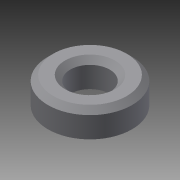
# Autodesk Inventor part: SpoolHandle-stop1
Saved by Autodesk Inventor 2014 (Build 180170000, 170)
## iProperties
Created: 2014-04-05
Part Number: SpoolHandle-stop1
Material: Generic
Document SubType Name: Modeling
Designer: Krzysiek
Density: 1 g/cm^3
Appearance: Default
Author: Krzysiek
Autodesk Inventor part; units mm, degrees
ref_plane "YZ Plane" through (0, 0, 0) normal (1, 0, 0) x (0, 1, 0)
ref_plane "XZ Plane" through (0, 0, 0) normal (0, 1, 0) x (-1, 0, 0)
ref_plane "XY Plane" through (0, 0, 0) normal (0, 0, 1) x (1, 0, 0)
sketch "Sketch1" plane through (0, 0, 0) normal (0, 0, 1) x (1, 0, 0)
  circle A0 centre (0, 0) radius 8
  dimension "d0" = 16
  constraints: 1 centre point, 1 coincident
  measures "d0" diameter of A0
extrude "Extrusion1" add sketch "Sketch1" along normal blind 5
sketch "Sketch2" plane through (0, 0, 5) normal (0, 0, 1) x (1, 0, 0)
  circle A0 centre (0, 0) radius 8 projected
  circle A1 centre (0, 0) radius 3.75
  dimension "d3" = 7.5
  constraints: 1 centre point, 1 coincident
  measures "d3" diameter of A1
extrude "Extrusion2" cut sketch "Sketch2" against normal blind 5 contours A1
chamfer "Chamfer1" distance 1 angle 45 1 edges at (-3.75, 0, 5)
chamfer "Chamfer2" distance 1 angle 45 1 edges at (-8, 0, 5)
body "Solid1"
